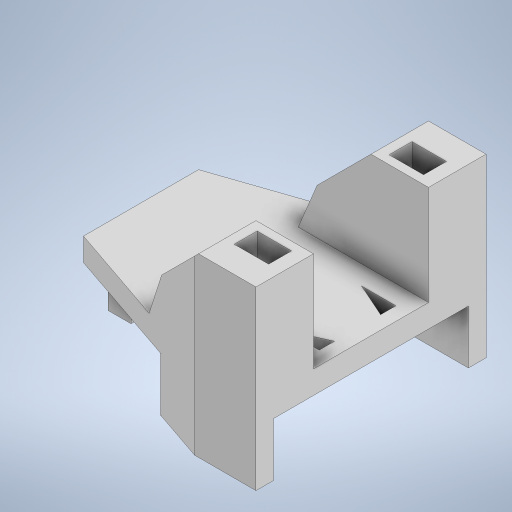
# Autodesk Inventor part: IRMount_top
Saved by Autodesk Inventor 2024.2 (Build 282272000, 272)
## iProperties
Created: 2024-04-04
Part Number: IRMount_top
Material: Generic
Document SubType Name: Modeling
Designer: ringl
Density: 1 g/cm^3
Appearance: Default
Author: ringl
Autodesk Inventor part; units mm, degrees
ref_plane "YZ Plane" through (0, 0, 0) normal (1, 0, 0) x (0, 1, 0)
ref_plane "XZ Plane" through (0, 0, 0) normal (0, 1, 0) x (-1, 0, 0)
ref_plane "XY Plane" through (0, 0, 0) normal (0, 0, 1) x (1, 0, 0)
sketch "Sketch1" plane through (0, 0, 0) normal (0, 1, 0) x (-1, 0, 0)
  line L0 (0, 0) -> (8, 0)
  line L1 (8, -30) -> (0, -30)
  line L2 (0, -30) -> (0, 0)
  line L3 (6.25, -3.4) -> (1.75, -3.4)
  line L4 (1.75, -3.4) -> (1.75, -6.4)
  line L5 (1.75, -6.4) -> (6.25, -6.4)
  line L6 (6.25, -6.4) -> (6.25, -3.4)
  line L7 (6.25, -23.6) -> (1.75, -23.6)
  line L8 (1.75, -23.6) -> (1.75, -26.6)
  line L9 (1.75, -26.6) -> (6.25, -26.6)
  line L10 (6.25, -26.6) -> (6.25, -23.6)
  line L11 (8, 0) -> (30, -7.5)
  line L12 (30, -7.5) -> (30, -22.5)
  line L13 (30, -22.5) -> (8, -30)
  dimension "d0" = 30
  dimension "d1" = 8
  dimension "d2" = 4.5
  dimension "d3" = 3
  dimension "d4" = 3
  dimension "d5" = 17.2
  dimension "d6" = 3.4
  dimension "d7" = 1.75
  dimension "d8" = 15
  dimension "d9" = 7.5
  dimension "d10" = 22
  dimension "d11" = 22
  constraints: 28 end point, 5 parallel, 3 horizontal, 2 perpendicular, 2 point on line, 1 coincident, 1 vertical
  measures "d0" distance between parallel lines of L0 L1
  measures "d1" distance of L1.start L1.end
  measures "d2" distance of L5.start L5.end
  measures "d3" distance of L3.end L5.start
  measures "d4" distance of L7.end L8.end
  measures "d5" distance between parallel lines of L7 L5
  measures "d6" distance between parallel lines of L0 L3
  measures "d7" distance between parallel lines of L2 L8
  measures "d8" distance of L11.end L12.end
  measures "d9" vertical distance of L0.end L11.end
  measures "d10" distance from line of L1.start L12
  measures "d11" horizontal distance of L0.end L11.end
extrude "Extrusion1" add sketch "Sketch1" along normal blind 3
sketch "Sketch2" plane through (0, 0, 0) normal (0, -1, 0) x (1, 0, 0)
  line L0 (0, -30) -> (-8, -30) projected
  line L1 (0, -30) -> (-8, -30)
  line L2 (-8, -30) -> (-14.7467, -27.7)
  line L3 (-8, -30) -> (-30, -22.5) projected
  line L4 (-14.7467, -27.7) -> (0, -27.7)
  line L5 (0, 0) -> (0, -30) projected
  line L6 (0, -27.7) -> (0, -30)
  line L7 (-14.7467, -2.3) -> (-8, 0)
  line L8 (-8, 0) -> (0, 0)
  line L9 (-14.7467, -2.3) -> (0, -2.3)
  line L10 (0, 0) -> (0, -2.3)
  dimension "d14" = 2.3
  dimension "d15" = 2.3
  dimension "d26" = 14.7467
  constraints: 16 end point, 2 collinear, 2 horizontal, 2 perpendicular, 2 point on line
  measures "d14" distance between parallel lines of L8 L9
  measures "d15" distance between parallel lines of L0 L4
  measures "d26" horizontal distance of L5.start L7.start
extrude "Extrusion2" add sketch "Sketch2" along normal blind 7
sketch "Sketch3" plane through (0, 0, 0) normal (0, -1, 0) x (1, 0, 0)
  line L0 (-27, -22.3) -> (-24, -22.3)
  line L1 (-24, -22.3) -> (-24, -7.7)
  line L2 (-24, -7.7) -> (-27, -7.7)
  line L3 (-27, -7.7) -> (-27, -22.3)
  line L4 (0, -2.3) -> (0, -27.7) projected
  circle A0 centre (-7, -15) radius 1.4
  circle A1 centre (-7, -15) radius 2
  line L5 (-8, -30) -> (0, -30) projected
  point P0 (0, 0)
  point P1 (-30, -7.5)
  point P2 (-30, -22.5)
  dimension "d27" = 3
  dimension "d28" = 24
  dimension "d29" = 14.6
  dimension "d30" = 0.2
  dimension "d31" = 2.8
  dimension "d32" = 4
  dimension "d33" = 7
  dimension "d34" = 15
  constraints: 8 end point, 2 centre point, 2 parallel, 1 coincident, 1 horizontal, 1 perpendicular
  measures "d27" distance of L1.end L2.end
  measures "d28" distance between parallel lines of L4 L1
  measures "d29" distance of L0.end L1.end
  measures "d30" distance from line of point (-30, -7.5) L2
  measures "d31" diameter of A0
  measures "d32" diameter of A1
  measures "d33" distance from line of L4 A0.centre
  measures "d34" distance from line of L5 A0.centre
extrude "Extrusion3" add sketch "Sketch3" along normal blind 4
fillet "Fillet1" radius 2 1 edges at (-9, 0, -15)
sketch "Sketch4" plane through (0, 3, 0) normal (0, 1, 0) x (1, 0, 0)
  circle A0 centre (-7, 15) radius 2 projected
  circle A1 centre (-7, 15) radius 1.4 projected
  circle A2 centre (-7, 15) radius 4 projected
  line L0 (-1.75, 10) -> (-6.25, 10)
  line L1 (-6.25, 10) -> (-1.75, 12)
  line L2 (-1.75, 10) -> (-1.75, 12)
  line L3 (-1.75, 18) -> (-1.75, 20)
  line L4 (-1.75, 20) -> (-6.25, 20)
  line L5 (-6.25, 20) -> (-1.75, 18)
  point P0 (0, 0)
  point P1 (-6.25, 6.4)
  point P2 (-1.75, 6.4)
  point P3 (-6.25, 23.6)
  point P4 (-1.75, 23.6)
  dimension "d38" = 3
  dimension "d39" = 2
  dimension "d40" = 2
  dimension "d41" = 3
  constraints: 12 end point, 4 vertical alignment, 2 vertical, 1 horizontal, 1 perpendicular
  measures "d38" vertical distance of L1.end A0.centre
  measures "d39" distance of L0.start L1.end
  measures "d40" distance of L3.start L3.end
  measures "d41" vertical distance of A0.centre L3.start
extrude "Extrusion4" cut sketch "Sketch4" against normal blind 5 contours L0 L1 L2 | L5 L4 L3
sketch "Sketch5" plane through (0, 3, 0) normal (0, 1, 0) x (1, 0, 0)
  circle A0 centre (-15.5, 17.5) radius 3
  line L0 (0, 0) -> (0, 30) projected
  point P0 (-30, 22.5)
  dimension "d44" = 6
  dimension "d45" = 15.5
  dimension "d46" = 5
  constraints: 1 centre point
  measures "d44" diameter of A0
  measures "d45" distance from line of L0 A0.centre
  measures "d46" vertical distance of point (-30, 22.5) A0.centre
extrude "Extrusion5" cut sketch "Sketch5" against normal blind 5
sketch "Sketch6" plane through (0, 3, 0) normal (0, 1, 0) x (1, 0, 0)
  line L0 (-6.25, 26.6) -> (-1.75, 26.6) projected
  line L1 (-1.75, 23.6) -> (-6.25, 23.6) projected
  line L2 (-6.25, 26.6) -> (-1.75, 26.6)
  line L3 (-1.75, 26.6) -> (-1.75, 23.6)
  line L4 (-1.75, 23.6) -> (-6.25, 23.6)
  line L5 (-6.25, 23.6) -> (-6.25, 26.6)
  line L6 (-6.25, 6.4) -> (-1.75, 6.4) projected
  line L7 (-6.25, 6.4) -> (-1.75, 6.4)
  line L8 (-1.75, 6.4) -> (-1.75, 3.4)
  line L9 (-1.75, 3.4) -> (-6.25, 3.4)
  line L10 (-6.25, 3.4) -> (-6.25, 6.4)
  line L11 (-8, 0) -> (0, 0) projected
  line L12 (0, 0) -> (-8, 0)
  line L13 (0, 0) -> (0, 30) projected
  line L14 (0, 7.5) -> (0, 0)
  line L15 (0, 30) -> (-8, 30)
  line L16 (0, 22.5) -> (0, 30)
  line L17 (-8, 30) -> (-30, 22.5) projected
  line L18 (-8, 30) -> (-17, 26.9318)
  line L19 (0, 22.5) -> (-17, 22.5)
  line L20 (-17, 26.9318) -> (-17, 22.5)
  line L21 (-8, 0) -> (-17, 3.0682)
  line L22 (-30, 7.5) -> (-8, 0) projected
  line L23 (-17, 3.0682) -> (-17, 7.5)
  line L24 (-17, 7.5) -> (0, 7.5)
  dimension "d52" = 3
  dimension "d55" = 17
  dimension "d56" = 1.1
  dimension "d57" = 17
  dimension "d58" = 1.1
  constraints: 36 end point, 5 point on line, 4 horizontal, 4 parallel, 3 perpendicular, 2 vertical, 1 collinear
  measures "d52" distance of L7.end L8.end
  measures "d55" distance of L16.start L19.end
  measures "d56" distance between parallel lines of L1 L19
  measures "d57" distance between parallel lines of L14 L23
  measures "d58" distance between parallel lines of L6 L24
extrude "Extrusion7" add sketch "Sketch6" along normal blind 13
chamfer "Chamfer1" distance 9.5 angle 45 2 edges at (-17, 16, -24.7159) (-17, 16, -5.2841)
chamfer "Chamfer2" distance 3.5 angle 45 2 edges at (-17, 6.5, -5.2841) (-17, 6.5, -24.7159)
body "Solid1"
